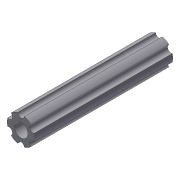
# Autodesk Inventor part: HopperPlateOffset
Saved by Autodesk Inventor 2012 (Build 160160000, 160)
## iProperties
Created: 2013-01-23
Part Number: HopperPlateOffset
Material: Aluminum-6061
Document SubType Name: Modeling
Designer: JesseK
Mass: 16.3494 g
Surface Area: 39.9032 cm^2
Volume: 6.03299 cm^3
Density: 2.71 g/cm^3
Author: JesseK
Autodesk Inventor part; units mm, degrees
ref_plane "YZ Plane" through (0, 0, 0) normal (1, 0, 0) x (0, 1, 0)
ref_plane "XZ Plane" through (0, 0, 0) normal (0, 1, 0) x (-1, 0, 0)
ref_plane "XY Plane" through (0, 0, 0) normal (0, 0, 1) x (1, 0, 0)
sketch "Sketch1" plane through (0, 0, 0) normal (0, 0, 1) x (1, 0, 0)
  circle A0 centre (0, 0) radius 3.175
  circle A1 centre (0, 0) radius 6.35
  dimension "d0" = 12.7
  dimension "d1" = 6.35
  constraints: 2 centre point, 2 coincident
  measures "d0" diameter of A1
  measures "d1" diameter of A0
extrude "Extrusion1" add sketch "Sketch1" along normal blind 63.5
sketch "Sketch2" plane through (0, 0, 0) normal (0, 0, -1) x (-1, 0, 0)
  circle A0 centre (0, 0) radius 6.35 projected
  arc A1 (-1.575, 6.1516) -> (1.575, 6.1516) centre (0, 6.35) ccw
  line L0 (0, 6.35) -> (0, 0) construction
  arc A2 (1.575, 6.1516) -> (-1.575, 6.1516) centre (0, 0) ccw
  dimension "d4" = 1.5875
  constraints: 7 point on circle, 2 centre point, 2 end point, 1 coincident, 1 vertical
  measures "d4" radius of A1
extrude "Extrusion2" cut sketch "Sketch2" against normal through all contours A1 A0 picked at (0, 5.8061)
pattern_circular "Circular Pattern1" count 6 over 360 about axis through (0, 0, 0) along (0, 0, 1) of "Extrusion2"
body "Solid1"
